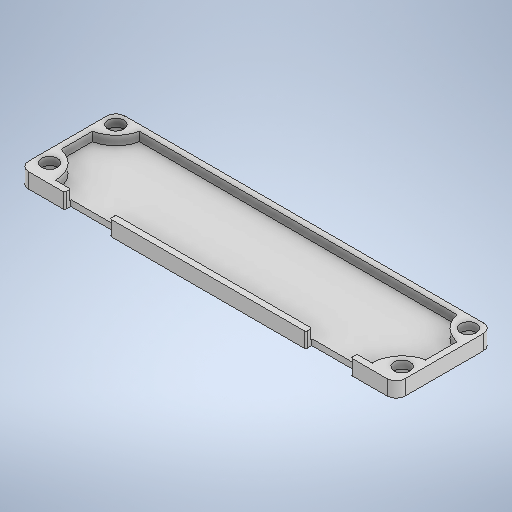
# Autodesk Inventor part: NozzleBoxLid
Saved by Autodesk Inventor 2025 (Build 290162000, 162)
## iProperties
Created: 2025-03-05
Part Number: NozzleBoxLid
Material: Типовые
Document SubType Name: Modeling
Designer: Makusimu
Density: 1 g/cm^3
Appearance: По умолчанию
Author: Makusimu
Autodesk Inventor part; units mm, degrees
ref_plane "YZ Plane" through (0, 0, 0) normal (1, 0, 0) x (0, 1, 0)
ref_plane "XZ Plane" through (0, 0, 0) normal (0, 1, 0) x (-1, 0, 0)
ref_plane "XY Plane" through (0, 0, 0) normal (0, 0, 1) x (1, 0, 0)
sketch "Эскиз1" plane through (0, 0, 0) normal (0, 1, 0) x (-1, 0, 0)
  line L0 (0, 0) -> (125, 0)
  line L1 (125, 0) -> (125, -32)
  line L2 (125, -32) -> (0, -32)
  line L3 (0, -32) -> (0, 0)
  dimension "d0" = 125
  dimension "d1" = 32
  constraints: 8 end point, 2 parallel, 1 horizontal, 1 perpendicular
  measures "d0" distance of L1.end L2.end
  measures "d1" distance of L0.end L1.end
extrude "Выдавливание1" add sketch "Эскиз1" along normal blind 5
sketch "Эскиз2" plane through (0, 5, 0) normal (0, 1, 0) x (1, 0, 0)
  line L0 (-2, 2) -> (-123, 2)
  line L1 (-123, 2) -> (-123, 30)
  line L2 (-123, 30) -> (-2, 30)
  line L3 (-2, 30) -> (-2, 2)
  line L4 (-125, 0) -> (0, 0) projected
  line L5 (-125, 32) -> (-125, 0) projected
  line L6 (0, 32) -> (-125, 32) projected
  line L7 (0, 0) -> (0, 32) projected
  arc A0 (-125, 22) -> (-115, 32) centre (-125, 32) ccw
  arc A1 (-10, 32) -> (0, 22) centre (0, 32) ccw
  arc A2 (0, 12) -> (-10, 2) centre (0, 2) ccw
  arc A3 (-115, 2) -> (-125, 12) centre (-125, 2) ccw
  point P0 (-2, 22.202)
  point P1 (-9.798, 30)
  point P2 (-115.202, 30)
  point P3 (-123, 22.202)
  point P4 (-123, 11.798)
  point P5 (-2, 11.798)
  dimension "d6" = 2
  dimension "d7" = 2
  dimension "d8" = 2
  dimension "d9" = 2
  dimension "d10" = 10
  dimension "d13" = 10
  dimension "d43" = 10
  constraints: 10 point on line, 8 end point, 8 point on circle, 4 centre point, 2 coincident, 2 parallel, 1 horizontal, 1 perpendicular
  measures "d6" distance between parallel lines of L4 L0
  measures "d7" distance between parallel lines of L5 L1
  measures "d8" distance between parallel lines of L6 L2
  measures "d9" distance between parallel lines of L7 L3
  measures "d10" radius of A0
  measures "d13" radius of A1
  measures "d43" radius of A2
extrude "Выдавливание2" cut sketch "Эскиз2" against normal blind 3 contours L0 A3 L1 A0 L2 A1 L3 A2
sketch "Эскиз3" plane through (0, 5, 0) normal (0, 1, 0) x (1, 0, 0)
  circle A0 centre (-121, 28) radius 2.65
  circle A1 centre (-121, 6) radius 2.65
  circle A2 centre (-4, 6) radius 2.65
  circle A3 centre (-4, 28) radius 2.65
  line L0 (0, 32) -> (-125, 32) projected
  line L1 (-125, 32) -> (-125, 0) projected
  line L2 (-125, 0) -> (0, 0) projected
  line L3 (0, 0) -> (0, 32) projected
  dimension "d16" = 5.3
  dimension "d17" = 5.3
  dimension "d18" = 5.3
  dimension "d19" = 5.3
  dimension "d20" = 4
  dimension "d21" = 4
  dimension "d22" = 4
  dimension "d23" = 6
  dimension "d24" = 6
  dimension "d25" = 4
  dimension "d26" = 4
  dimension "d27" = 4
  constraints: 4 centre point
  measures "d16" diameter of A0
  measures "d17" diameter of A1
  measures "d18" diameter of A2
  measures "d19" diameter of A3
  measures "d20" distance from line of L0 A0.centre
  measures "d21" distance from line of L1 A0.centre
  measures "d22" distance from line of L1 A1.centre
  measures "d23" distance from line of L2 A1.centre
  measures "d24" distance from line of L2 A2.centre
  measures "d25" distance from line of L3 A2.centre
  measures "d26" distance from line of L0 A3.centre
  measures "d27" distance from line of L3 A3.centre
extrude "Выдавливание3" cut sketch "Эскиз3" against normal blind 2.6 contours A0 | A1 | A2 | A3
sketch "Эскиз4" plane through (-125, 0, 0) normal (0, 0, 1) x (1, 0, 0)
  line L0 (125, 0) -> (0, 0) projected
  line L1 (125, 5) -> (0, 5) projected
  line L2 (15, 0) -> (30, 0)
  line L3 (30, 0) -> (30, 5)
  line L4 (30, 5) -> (15, 5)
  line L5 (15, 5) -> (15, 0)
  line L6 (95, 5) -> (110, 5)
  line L7 (110, 5) -> (110, 0)
  line L8 (110, 0) -> (95, 0)
  line L9 (95, 0) -> (95, 5)
  line L10 (0, 0) -> (0, 5) projected
  line L11 (125, 0) -> (125, 5) projected
  point P0 (110, 0)
  dimension "d32" = 15
  dimension "d33" = 30
  dimension "d34" = 15
  dimension "d35" = 30
  constraints: 16 end point, 4 parallel, 4 point on line, 2 horizontal, 2 perpendicular
  measures "d32" distance between parallel lines of L10 L5
  measures "d33" distance between parallel lines of L10 L3
  measures "d34" distance between parallel lines of L11 L7
  measures "d35" distance between parallel lines of L11 L9
extrude "Выдавливание4" cut sketch "Эскиз4" against normal blind 2 contours L0 L9 L1 L7 | L0 L5 L1 L3
fillet "Сопряжение2" radius 3 4 edges at (-125, 2.5, 0) (0, 2.5, 0) (0, 2.5, -32) (-125, 2.5, -32)
fillet "Сопряжение4" radius 0.5 8 edges at (-110, 2.5, 0) (-95, 2.5, 0) (-30, 2.5, 0) (-15, 2.5, 0) (-110, 3.5, -2) (-95, 3.5, -2) (-30, 3.5, -2) (-15, 3.5, -2)
sketch "Эскиз5" plane through (0, 0, 0) normal (0, -1, 0) x (1, 0, 0)
  line L0 (-105.8351, -8.1135) -> (-33.1329, -8.1135) construction
  line L1 (-33.1329, -8.1135) -> (-33.1329, -24.0837) construction
  line L2 (-33.1329, -24.0837) -> (-105.8351, -24.0837) construction
  line L3 (-105.8351, -24.0837) -> (-105.8351, -8.1135) construction
  line L4 (-97.9947, -23.1135) -> (-100.4008, -23.1135)
  line L5 (-100.4008, -23.1135) -> (-100.8351, -10.5782)
  line L6 (-100.8351, -10.5782) -> (-102.7951, -23.1135)
  line L7 (-102.7951, -23.1135) -> (-105.0721, -23.1135)
  line L8 (-105.0721, -23.1135) -> (-102.5017, -8.1135)
  line L9 (-102.5017, -8.1135) -> (-98.8984, -8.1135)
  line L10 (-98.8984, -8.1135) -> (-98.5228, -18.6182)
  line L11 (-98.5228, -18.6182) -> (-94.3797, -8.1135)
  line L12 (-94.3797, -8.1135) -> (-90.7177, -8.1135)
  line L13 (-90.7177, -8.1135) -> (-93.2529, -23.1135)
  line L14 (-93.2529, -23.1135) -> (-95.5651, -23.1135)
  line L15 (-95.5651, -23.1135) -> (-93.1825, -10.6721)
  line L16 (-93.1825, -10.6721) -> (-97.9947, -23.1135)
  line L17 (-87.443, -15.3318) -> (-89.7905, -15.0853)
  spline S0 degree 2 poles (-89.7905, -15.0853) (-89.3679, -13.5829) (-87.2905, -11.9984) (-85.6942, -11.9984) knots 0 0 0 1 2 2 2
  spline S1 degree 2 poles (-85.6942, -11.9984) (-84.0628, -11.9984) (-82.3139, -13.6064) (-82.3139, -14.9444) knots 0 0 0 1 2 2 2
  spline S2 degree 2 poles (-82.3139, -14.9444) (-82.3139, -15.4139) (-82.4782, -16.4703) (-83.0064, -18.8294) knots 0 0 0 1 2 2 2
  spline S3 degree 2 poles (-83.0064, -18.8294) (-83.4524, -20.7778) (-83.4524, -21.5524) knots 0 0 0 1 1 1
  spline S4 degree 2 poles (-83.4524, -21.5524) (-83.4524, -22.2684) (-83.2059, -23.1135) knots 0 0 0 1 1 1
  line L18 (-83.2059, -23.1135) -> (-85.612, -23.1135)
  spline S5 degree 2 poles (-85.612, -23.1135) (-85.7529, -22.5149) (-85.7881, -21.8811) knots 0 0 0 1 1 1
  spline S6 degree 2 poles (-85.7881, -21.8811) (-86.3045, -22.597) (-87.6308, -23.3599) (-88.2881, -23.3599) knots 0 0 0 1 2 2 2
  spline S7 degree 2 poles (-88.2881, -23.3599) (-89.3327, -23.3599) (-90.7529, -21.6463) (-90.7529, -20.2027) knots 0 0 0 1 2 2 2
  spline S8 degree 2 poles (-90.7529, -20.2027) (-90.7529, -18.5595) (-89.9196, -17.6674) knots 0 0 0 1 1 1
  spline S9 degree 2 poles (-89.9196, -17.6674) (-89.0862, -16.7754) (-87.1379, -16.5994) knots 0 0 0 1 1 1
  spline S10 degree 2 poles (-87.1379, -16.5994) (-85.4125, -16.4233) (-84.8374, -16.1768) knots 0 0 0 1 1 1
  spline S11 degree 2 poles (-84.8374, -16.1768) (-84.6379, -15.5548) (-84.6379, -15.1909) knots 0 0 0 1 1 1
  spline S12 degree 2 poles (-84.6379, -15.1909) (-84.6379, -14.698) (-85.3186, -14.0876) (-85.8937, -14.0876) knots 0 0 0 1 2 2 2
  spline S13 degree 2 poles (-85.8937, -14.0876) (-87.1613, -14.0876) (-87.443, -15.3318) knots 0 0 0 1 1 1
  spline S14 degree 2 poles (-85.2247, -18.0548) (-85.4477, -18.1252) (-85.7998, -18.1839) knots 0 0 0 1 1 1
  spline S15 degree 2 poles (-85.7998, -18.1839) (-87.443, -18.4304) (-88.4876, -19.2637) (-88.4876, -19.9562) knots 0 0 0 1 2 2 2
  spline S16 degree 2 poles (-88.4876, -19.9562) (-88.4876, -20.4961) (-87.889, -21.1651) (-87.4313, -21.1651) knots 0 0 0 1 2 2 2
  spline S17 degree 2 poles (-87.4313, -21.1651) (-86.9618, -21.1651) (-86.0815, -20.6017) (-85.5651, -19.5923) (-85.3186, -18.4421) knots 0 0 0 1 2 3 3 3
  line L19 (-85.3186, -18.4421) -> (-85.2247, -18.0548)
  line L20 (-81.3163, -23.1135) -> (-78.7459, -8.1135)
  line L21 (-78.7459, -8.1135) -> (-76.328, -8.1135)
  line L22 (-76.328, -8.1135) -> (-77.666, -15.8834)
  line L23 (-77.666, -15.8834) -> (-74.544, -12.2449)
  line L24 (-74.544, -12.2449) -> (-71.4219, -12.2449)
  line L25 (-71.4219, -12.2449) -> (-75.0017, -16.1768)
  line L26 (-75.0017, -16.1768) -> (-73.0886, -23.1135)
  line L27 (-73.0886, -23.1135) -> (-75.5064, -23.1135)
  line L28 (-75.5064, -23.1135) -> (-76.7271, -18.0665)
  line L29 (-76.7271, -18.0665) -> (-78.3351, -19.8388)
  line L30 (-78.3351, -19.8388) -> (-78.8984, -23.1135)
  line L31 (-78.8984, -23.1135) -> (-81.3163, -23.1135)
  line L32 (-70.0604, -12.2449) -> (-67.6426, -12.2449)
  line L33 (-67.6426, -12.2449) -> (-68.7459, -18.6534)
  spline S18 degree 2 poles (-68.7459, -18.6534) (-68.9454, -19.8153) (-68.9454, -20.1088) knots 0 0 0 1 1 1
  spline S19 degree 2 poles (-68.9454, -20.1088) (-68.9454, -20.6017) (-68.3703, -21.2707) (-67.9477, -21.2707) knots 0 0 0 1 2 2 2
  spline S20 degree 2 poles (-67.9477, -21.2707) (-67.4665, -21.2707) (-66.9853, -20.9186) knots 0 0 0 1 1 1
  spline S21 degree 2 poles (-66.9853, -20.9186) (-66.3163, -20.4374) (-65.5182, -18.8998) (-65.2482, -17.421) knots 0 0 0 1 2 2 2
  line L34 (-65.2482, -17.421) -> (-64.274, -12.2449)
  line L35 (-64.274, -12.2449) -> (-61.8562, -12.2449)
  line L36 (-61.8562, -12.2449) -> (-63.875, -23.1135)
  line L37 (-63.875, -23.1135) -> (-66.1402, -23.1135)
  line L38 (-66.1402, -23.1135) -> (-65.8703, -21.6346)
  spline S22 degree 2 poles (-65.8703, -21.6346) (-67.3374, -23.3599) (-69.051, -23.3599) knots 0 0 0 1 1 1
  spline S23 degree 2 poles (-69.051, -23.3599) (-70.1191, -23.3599) (-71.3867, -21.8576) (-71.3867, -20.5313) knots 0 0 0 1 2 2 2
  spline S24 degree 2 poles (-71.3867, -20.5313) (-71.3867, -19.9797) (-71.105, -18.3012) knots 0 0 0 1 1 1
  line L39 (-71.105, -18.3012) -> (-70.0604, -12.2449)
  line L40 (-61.551, -20.0736) -> (-59.2153, -19.6275)
  spline S25 degree 2 poles (-59.2153, -19.6275) (-58.9102, -20.543) (-57.9712, -21.2707) (-57.1848, -21.2707) knots 0 0 0 1 2 2 2
  spline S26 degree 2 poles (-57.1848, -21.2707) (-56.4454, -21.2707) (-55.5182, -20.5548) (-55.5182, -20.0736) knots 0 0 0 1 2 2 2
  spline S27 degree 2 poles (-55.5182, -20.0736) (-55.5182, -19.7449) (-55.7177, -19.5219) knots 0 0 0 1 1 1
  spline S28 degree 2 poles (-55.7177, -19.5219) (-55.9172, -19.3106) (-56.6919, -19.0055) knots 0 0 0 1 1 1
  spline S29 degree 2 poles (-56.6919, -19.0055) (-58.8632, -18.1369) (-59.3797, -17.6322) knots 0 0 0 1 1 1
  spline S30 degree 2 poles (-59.3797, -17.6322) (-60.213, -16.8224) (-60.213, -15.5196) knots 0 0 0 1 1 1
  spline S31 degree 2 poles (-60.213, -15.5196) (-60.213, -13.982) (-58.0416, -11.9984) (-56.1637, -11.9984) knots 0 0 0 1 2 2 2
  spline S32 degree 2 poles (-56.1637, -11.9984) (-52.9712, -11.9984) (-52.4548, -14.8388) knots 0 0 0 1 1 1
  line L41 (-52.4548, -14.8388) -> (-54.6731, -15.3083)
  spline S33 degree 2 poles (-54.6731, -15.3083) (-55.0604, -14.0172) (-56.5393, -14.0172) knots 0 0 0 1 1 1
  spline S34 degree 2 poles (-56.5393, -14.0172) (-57.2318, -14.0172) (-57.9477, -14.5923) (-57.9477, -15.0266) knots 0 0 0 1 2 2 2
  spline S35 degree 2 poles (-57.9477, -15.0266) (-57.9477, -15.4022) (-57.666, -15.6604) knots 0 0 0 1 1 1
  spline S36 degree 2 poles (-57.666, -15.6604) (-57.4665, -15.8482) (-56.2576, -16.2825) knots 0 0 0 1 1 1
  spline S37 degree 2 poles (-56.2576, -16.2825) (-54.5322, -16.9045) (-53.9336, -17.4797) knots 0 0 0 1 1 1
  spline S38 degree 2 poles (-53.9336, -17.4797) (-53.0651, -18.3365) (-53.0651, -19.5454) knots 0 0 0 1 1 1
  spline S39 degree 2 poles (-53.0651, -19.5454) (-53.0651, -21.1886) (-55.2951, -23.3599) (-57.1379, -23.3599) knots 0 0 0 1 2 2 2
  spline S40 degree 2 poles (-57.1379, -23.3599) (-60.7646, -23.3599) (-61.551, -20.0736) knots 0 0 0 1 1 1
  line L42 (-49.8139, -12.2449) -> (-47.4078, -12.2449)
  line L43 (-47.4078, -12.2449) -> (-49.2623, -23.1135)
  line L44 (-49.2623, -23.1135) -> (-51.6801, -23.1135)
  line L45 (-51.6801, -23.1135) -> (-49.8139, -12.2449)
  line L46 (-49.1097, -8.1135) -> (-46.6919, -8.1135)
  line L47 (-46.6919, -8.1135) -> (-47.1496, -10.766)
  line L48 (-47.1496, -10.766) -> (-49.5557, -10.766)
  line L49 (-49.5557, -10.766) -> (-49.1097, -8.1135)
  line L50 (-45.2365, -12.2449) -> (-42.9477, -12.2449)
  line L51 (-42.9477, -12.2449) -> (-43.1825, -13.5595)
  spline S41 degree 2 poles (-43.1825, -13.5595) (-41.8327, -11.9984) (-40.3538, -11.9984) knots 0 0 0 1 1 1
  spline S42 degree 2 poles (-40.3538, -11.9984) (-38.382, -11.9984) (-38.0651, -13.9116) knots 0 0 0 1 1 1
  spline S43 degree 2 poles (-38.0651, -13.9116) (-37.5839, -13.0782) (-35.8233, -11.9984) (-34.9313, -11.9984) knots 0 0 0 1 2 2 2
  spline S44 degree 2 poles (-34.9313, -11.9984) (-33.875, -11.9984) (-32.6308, -13.3482) (-32.6308, -14.5454) knots 0 0 0 1 2 2 2
  spline S45 degree 2 poles (-32.6308, -14.5454) (-32.6308, -15.1088) (-32.8656, -16.482) knots 0 0 0 1 1 1
  line L52 (-32.8656, -16.482) -> (-34.0041, -23.1135)
  line L53 (-34.0041, -23.1135) -> (-36.4219, -23.1135)
  line L54 (-36.4219, -23.1135) -> (-35.2834, -16.4703)
  spline S46 degree 2 poles (-35.2834, -16.4703) (-35.0721, -15.2261) (-35.0721, -15.0618) knots 0 0 0 1 1 1
  spline S47 degree 2 poles (-35.0721, -15.0618) (-35.0721, -14.5923) (-35.5534, -14.0876) (-35.9642, -14.0876) knots 0 0 0 1 2 2 2
  spline S48 degree 2 poles (-35.9642, -14.0876) (-36.8562, -14.0876) (-37.5604, -15.1674) knots 0 0 0 1 1 1
  spline S49 degree 2 poles (-37.5604, -15.1674) (-38.1238, -16.0243) (-38.4994, -18.1721) knots 0 0 0 1 1 1
  line L55 (-38.4994, -18.1721) -> (-39.3444, -23.1135)
  line L56 (-39.3444, -23.1135) -> (-41.7623, -23.1135)
  line L57 (-41.7623, -23.1135) -> (-40.6355, -16.5407)
  spline S50 degree 2 poles (-40.6355, -16.5407) (-40.4477, -15.4139) (-40.4477, -15.0853) knots 0 0 0 1 1 1
  spline S51 degree 2 poles (-40.4477, -15.0853) (-40.4477, -14.6158) (-40.9524, -14.0876) (-41.3515, -14.0876) knots 0 0 0 1 2 2 2
  spline S52 degree 2 poles (-41.3515, -14.0876) (-41.8797, -14.0876) (-43.0182, -15.0853) (-43.3468, -16.036) knots 0 0 0 1 2 2 2
  spline S53 degree 2 poles (-43.3468, -16.036) (-43.5463, -16.5994) (-43.8163, -18.1252) knots 0 0 0 1 1 1
  line L58 (-43.8163, -18.1252) -> (-44.6848, -23.1135)
  line L59 (-44.6848, -23.1135) -> (-47.1027, -23.1135)
  line L60 (-47.1027, -23.1135) -> (-45.2365, -12.2449)
  line L61 (-29.9665, -12.2449) -> (-27.5487, -12.2449)
  line L62 (-27.5487, -12.2449) -> (-28.652, -18.6534)
  spline S54 degree 2 poles (-28.652, -18.6534) (-28.8515, -19.8153) (-28.8515, -20.1088) knots 0 0 0 1 1 1
  spline S55 degree 2 poles (-28.8515, -20.1088) (-28.8515, -20.6017) (-28.2764, -21.2707) (-27.8538, -21.2707) knots 0 0 0 1 2 2 2
  spline S56 degree 2 poles (-27.8538, -21.2707) (-27.3726, -21.2707) (-26.8914, -20.9186) knots 0 0 0 1 1 1
  spline S57 degree 2 poles (-26.8914, -20.9186) (-26.2224, -20.4374) (-25.4243, -18.8998) (-25.1543, -17.421) knots 0 0 0 1 2 2 2
  line L63 (-25.1543, -17.421) -> (-24.1801, -12.2449)
  line L64 (-24.1801, -12.2449) -> (-21.7623, -12.2449)
  line L65 (-21.7623, -12.2449) -> (-23.7811, -23.1135)
  line L66 (-23.7811, -23.1135) -> (-26.0463, -23.1135)
  line L67 (-26.0463, -23.1135) -> (-25.7764, -21.6346)
  spline S58 degree 2 poles (-25.7764, -21.6346) (-27.2435, -23.3599) (-28.9571, -23.3599) knots 0 0 0 1 1 1
  spline S59 degree 2 poles (-28.9571, -23.3599) (-30.0252, -23.3599) (-31.2928, -21.8576) (-31.2928, -20.5313) knots 0 0 0 1 2 2 2
  spline S60 degree 2 poles (-31.2928, -20.5313) (-31.2928, -19.9797) (-31.0111, -18.3012) knots 0 0 0 1 1 1
  line L68 (-31.0111, -18.3012) -> (-29.9665, -12.2449)
  point P0 (0, 0)
  constraints: 2 other
emboss "Рельеф1" sketch "Эскиз5" operation cut depth 0.2 direction (0, 1, 0)
